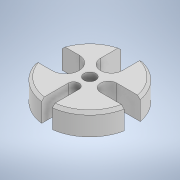
# Autodesk Inventor part: Ch7(5) Part 3 Table
Saved by Autodesk Inventor 2020 (Build 240168000, 168)
## iProperties
Created: 2021-02-25
Part Number: Ch7(5) Part 3 Table
Material: Generic
Document SubType Name: Modeling
Designer: adriggs
Density: 1 g/cm^3
Appearance: Default
Author: adriggs
Autodesk Inventor part; units mm, degrees
ref_plane "YZ Plane" through (0, 0, 0) normal (1, 0, 0) x (0, 1, 0)
ref_plane "XZ Plane" through (0, 0, 0) normal (0, 1, 0) x (-1, 0, 0)
ref_plane "XY Plane" through (0, 0, 0) normal (0, 0, 1) x (1, 0, 0)
sketch "Sketch1" plane through (0, 0, 0) normal (0, 1, 0) x (-1, 0, 0)
  line L0 (37.6078, 0) -> (-39.2505, 0) projected
  line L1 (0, -38.4978) -> (0, 39.9458) projected
  circle A0 centre (0, 0) radius 3.4798
  line L2 (3.1734, 25.201) -> (3.1734, 9.525)
  line L3 (-3.1734, 25.201) -> (-3.1734, 9.525)
  arc A1 (-3.1734, 9.525) -> (3.1734, 9.525) centre (0, 9.525) ccw
  line L4 (-6.35, -24.5934) -> (-6.35, -12.7)
  line L5 (6.35, -24.5934) -> (6.35, -12.7)
  arc A2 (6.35, -12.7) -> (-6.35, -12.7) centre (0, -12.7) ccw
  line L6 (-24.9495, 4.7625) -> (-11.0998, 4.7625)
  line L7 (-24.9495, -4.7625) -> (-11.0998, -4.7625)
  arc A3 (-11.0998, -4.7625) -> (-11.0998, 4.7625) centre (-11.0998, 0) ccw
  line L8 (24.1279, 7.9375) -> (14.2748, 7.9375)
  line L9 (24.1279, -7.9375) -> (14.2748, -7.9375)
  arc A4 (14.2748, 7.9375) -> (14.2748, -7.9375) centre (14.2748, 0) ccw
  arc A5 (-24.9495, -4.7625) -> (-6.35, -24.5934) centre (0, 0) ccw
  arc A6 (6.35, -24.5934) -> (24.1279, -7.9375) centre (0, 0) ccw
  arc A7 (24.1279, 7.9375) -> (3.1734, 25.201) centre (0, 0) ccw
  arc A8 (-3.1734, 25.201) -> (-24.9495, 4.7625) centre (0, 0) ccw
  dimension "d1" = 6.9596
  dimension "d5" = 9.525
  dimension "d6" = 12.7
  dimension "d7" = 9.525
  dimension "d8" = 6.3469
  dimension "d9" = 12.7
  dimension "d11" = 15.875
  dimension "d12" = 11.0998
  dimension "d13" = 14.2748
  dimension "d14" = 25.4
  constraints: 16 end point, 16 point on circle, 9 centre point, 7 vertical alignment, 6 horizontal alignment, 4 horizontal, 4 point on line, 4 vertical, 2 coincident, 2 concentric
  measures "d1" diameter of A0
  measures "d5" distance of A1.centre point (0, 0)
  measures "d6" distance of point (0, 0) A2.centre
  measures "d7" distance of L7.start L6.start
  measures "d8" distance of L3.start L2.start
  measures "d9" distance between parallel lines of L5 L4
  measures "d11" distance between parallel lines of L9 L8
  measures "d12" distance of point (0, 0) A3.centre
  measures "d13" distance of A4.centre point (0, 0)
  measures "d14" radius of A8
extrude "Extrusion1" add sketch "Sketch1" along normal blind 12.7 contours A4 L9 A6 L5 A2 L1 A0 L0 | L0 A0 L1 A1 L2 A7 L8 A4 | A0 L0 A3 L6 A8 L3 A1 L1 | L1 A2 L4 A5 L7 A3 L0 A0
chamfer "Chamfer1" distance 1.5875 angle 45 4 edges at (-16.1508, 12.7, 19.6039) (-17.3661, 12.7, -18.5359) (18.5265, 12.7, -17.3761) (17.3827, 12.7, 18.5203)
body "Solid1"
